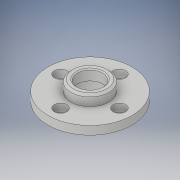
# Autodesk Inventor part: orczyk
Saved by Autodesk Inventor 2019 (Build 230136000, 136)
## iProperties
Created: 2021-10-14
Part Number: orczyk
Material: Generic
Document SubType Name: Modeling
Designer: Pokick
Density: 1 g/cm^3
Appearance: Default
Author: Pokick
Autodesk Inventor part; units mm, degrees
ref_plane "YZ Plane" through (0, 0, 0) normal (1, 0, 0) x (0, 1, 0)
ref_plane "XZ Plane" through (0, 0, 0) normal (0, 1, 0) x (-1, 0, 0)
ref_plane "XY Plane" through (0, 0, 0) normal (0, 0, 1) x (1, 0, 0)
sketch "Sketch1" plane through (0, 0, 0) normal (0, 1, 0) x (-1, 0, 0)
  circle A0 centre (0, 0) radius 10
  circle A1 centre (0, 0) radius 3.025
  circle A2 centre (0, 0) radius 7 construction
  line L0 (0, 0) -> (0, -10) construction
  circle A3 centre (0, -7) radius 1.5
  line L1 (0, 0) -> (10, 0) construction
  circle A4 centre (7, 0) radius 1.5
  line L2 (0, 0) -> (0, 10) construction
  circle A5 centre (0, 7) radius 1.5
  line L3 (0, 0) -> (-10, 0) construction
  circle A6 centre (-7, 0) radius 1.5
  dimension "d0" = 20
  dimension "d2" = 14
  dimension "d1" = 6.05
  dimension "d3" = 3
  dimension "d6" = 360
  constraints: 8 end point, 5 centre point, 4 point on line, 3 coincident, 2 vertical alignment, 1 vertical, 25 other
  measures "d1" diameter of A1
  measures "d3" diameter of A3
extrude "Extrusion1" add sketch "Sketch1" along normal blind 2
sketch "Sketch2" plane through (0, 2, 0) normal (0, 1, 0) x (1, 0, 0)
  circle A0 centre (0, 0) radius 3
  circle A1 centre (0, 0) radius 4.5
  dimension "d10" = 6
  dimension "d11" = 9
  constraints: 2 centre point, 2 coincident
  measures "d10" diameter of A0
  measures "d11" diameter of A1
extrude "Extrusion2" add sketch "Sketch2" along normal blind 2.5
chamfer "Chamfer1" distance 0.5 angle 45 1 edges at (-4.5, 4.5, 0)
chamfer "Chamfer2" distance 0.25 angle 45 1 edges at (-3, 4.5, 0)
body "Solid1"
